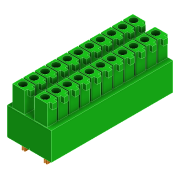
# Autodesk Inventor part: conectores_macho
Saved by Autodesk Inventor 2022 (Build 260153000, 153)
## iProperties
Created: 2022-11-18
Part Number: conectores_macho
Material: Generic
Document SubType Name: Modeling
Designer: ferna
Density: 1 g/cm^3
Appearance: Default
Author: ferna
Autodesk Inventor part; units mm, degrees
ref_plane "YZ Plane" through (0, 0, 0) normal (1, 0, 0) x (0, 1, 0)
ref_plane "XZ Plane" through (0, 0, 0) normal (0, 1, 0) x (-1, 0, 0)
ref_plane "XY Plane" through (0, 0, 0) normal (0, 0, 1) x (1, 0, 0)
sketch "Sketch1" plane through (0, 0, 0) normal (0, 1, 0) x (-1, 0, 0)
  line L0 (-4.4594, 3.5) -> (0, 3.5)
  line L1 (-4.4594, 2.5) -> (-4.4594, 3.5)
  line L2 (-4.6594, 2.5) -> (-4.4594, 2.5)
  line L3 (-4.6594, 2.8) -> (-4.6594, 2.5)
  line L4 (-6, 3.5) -> (-4.6594, 2.8)
  line L5 (-6, 0) -> (-6, 3.5)
  line L6 (-4.6594, 0.7) -> (-6, 0)
  line L7 (-4.6594, 1) -> (-4.6594, 0.7)
  line L8 (-4.4594, 1) -> (-4.6594, 1)
  line L9 (-4.4594, 0) -> (-4.4594, 1)
  line L10 (0, 0) -> (-4.4594, 0)
  line L11 (0, 3.5) -> (0, 0)
  line L12 (0.25, 0) -> (1.75, 0)
  line L13 (1.75, 3.5) -> (1.75, 0)
  line L14 (1.75, 3.5) -> (0.25, 3.5)
  line L15 (0.25, 0) -> (0.25, 3.5)
  line L16 (-6.25, 43.75) -> (-6.25, -0.25)
  line L17 (-2.2297, 3.75) -> (-6.25, 3.75)
  constraints: 36 end point, 1 perpendicular, 1 point on line
extrude "Extrusion1" add sketch "Sketch1" along normal blind 7.5 contours L0 L11 L10 L9 L8 L7 L6 L5 L4 L3 L2 L1
sketch "Sketch2" plane through (0, 7.5, 0) normal (0, 1, 0) x (1, 0, 0)
  line L0 (0, 0) -> (0, -3.5) projected
  line L1 (0, -1.75) -> (2, -1.75)
  circle A0 centre (2, -1.75) radius 1.3281
  dimension "d2" = 2
  constraints: 2 end point, 1 centre point, 1 coincident, 1 horizontal, 1 midpoint
  measures "d2" distance of L1.start L1.end
extrude "Extrusion2" cut sketch "Sketch2" against normal blind 7.5
sketch "Sketch3" plane through (0, 7.5, 0) normal (0, 1, 0) x (1, 0, 0)
  line L0 (4.6594, -2.5) -> (4.6594, -2.8) projected
  line L1 (4.6594, -2.5) -> (6.5607, -2.5)
  line L2 (6.5607, -2.5) -> (6.5607, -3.7591)
  line L3 (6.5607, -3.7591) -> (4.6594, -3.7591)
  line L4 (4.6594, -3.7591) -> (4.6594, -2.5)
  line L5 (4.6594, -1) -> (4.4594, -1) projected
  line L6 (4.6594, -1) -> (6.277, -1)
  line L7 (6.277, -1) -> (6.277, 0.4256)
  line L8 (6.277, 0.4256) -> (4.6594, 0.4256)
  line L9 (4.6594, 0.4256) -> (4.6594, -1)
  line L10 (5.61, -2.5) -> (6.277, -2.5)
  line L11 (6.277, -2.5) -> (6.277, -1)
  line L12 (6.277, -1) -> (5.61, -1)
  line L13 (5.61, -1) -> (5.61, -2.5)
  point P0 (0, 0)
  constraints: 24 end point, 6 parallel, 3 horizontal, 3 perpendicular, 1 midpoint
extrude "Extrusion3" cut sketch "Sketch3" against normal blind 7.5
sketch "Sketch4" plane through (5.61, 7.5, 2.5) normal (1, 0, 0) x (0, 0, -1)
  line L0 (0, -7.5) -> (0, 0) projected
  line L1 (0, -1.9796) -> (1.6962, -1.9796)
  line L2 (1.6962, -1.9796) -> (1.6962, -7.8428)
  line L3 (1.6962, -7.8428) -> (0, -7.8428)
  line L4 (0, -7.8428) -> (0, -1.9796)
  point P0 (2.5, -7.5)
  constraints: 8 end point, 2 parallel, 1 horizontal, 1 perpendicular, 1 point on line
extrude "Extrusion4" cut sketch "Sketch4" against normal up to surface (1.1506 mm away)
sketch "Sketch5" plane through (0, 0, 0) normal (0, -1, 0) x (1, 0, 0)
  line L0 (6.25, -40.25) -> (6.25, 3.75)
  line L1 (2.2297, -0.25) -> (6.25, -0.25)
  line L2 (-1.75, 0) -> (-1.75, 3.5)
  line L3 (4.4594, 0) -> (0, 0) projected
  line L4 (2.2297, 0) -> (2.2297, -0.25)
  line L5 (6.25, 3.75) -> (-1.75, 3.75)
  line L6 (0, 3.5) -> (4.4594, 3.5) projected
  line L7 (-1.75, 3.75) -> (-1.75, 3.5)
  line L8 (-1.75, 0) -> (-1.75, -0.25)
  line L9 (-1.75, -0.25) -> (2.2297, -0.25)
  dimension "d9" = 0.25
  constraints: 16 end point, 3 perpendicular, 2 point on line, 1 midpoint, 1 parallel, 1 vertical
  measures "d9" distance of L4.start L4.end
extrude "Extrusion5" add sketch "Sketch5" along normal blind 10
sketch "Sketch6" plane through (0, -10, 0) normal (0, -1, 0) x (1, 0, 0)
  line L0 (-1.75, 3.75) -> (-1.75, -0.25) projected
  line L1 (-1.75, -0.25) -> (-1.75, 1.75)
  line L2 (-1.75, 1.75) -> (0.25, 1.75)
  line L3 (0.25, 1.75) -> (4.25, 1.75)
  circle A0 centre (0.25, 1.75) radius 1.35
  line L4 (2.9, 0.4) -> (5.6, 0.4)
  line L5 (5.6, 0.4) -> (5.6, 3.1)
  line L6 (5.6, 3.1) -> (2.9, 3.1)
  line L7 (2.9, 3.1) -> (2.9, 0.4)
  line L8 (2.9, 0.4) -> (5.6, 3.1) construction
  line L9 (5.6, 0.4) -> (2.9, 3.1) construction
  point P0 (0, 0)
  dimension "d12" = 2
  dimension "d13" = 2
  dimension "d14" = 4
  dimension "d15" = 2.7
  dimension "d16" = 2.7
  dimension "d17" = 2.7
  constraints: 18 end point, 3 midpoint, 2 parallel, 2 perpendicular, 1 centre point, 1 coincident, 1 horizontal, 1 point on line
  measures "d12" distance of L0.end L1.end
  measures "d13" distance of L1.end L2.end
  measures "d14" distance of L2.end L3.end
  measures "d15" diameter of A0
  measures "d16" distance of L6.end L5.end
  measures "d17" distance of L5.end L4.end
extrude "Extrusion6" cut sketch "Sketch6" against normal blind 8
sketch "Sketch7" plane through (0, -2, 0) normal (0, -1, 0) x (1, 0, 0)
  line L0 (2.9, 3.1) -> (5.6, 3.1) projected
  line L1 (5.6, 0.4) -> (2.9, 0.4) projected
  line L2 (2.9, 3.1) -> (4.0783, 3.1)
  line L3 (4.0783, 3.1) -> (4.0783, 0.4)
  line L4 (4.0783, 0.4) -> (2.9, 0.4)
  line L5 (2.9, 0.4) -> (2.9, 3.1)
  point P0 (0, 0)
  constraints: 8 end point, 2 parallel, 1 horizontal, 1 perpendicular, 1 point on line
extrude "Extrusion7" add sketch "Sketch7" along normal blind 9 separate body
sketch "Sketch8" plane through (0, -11, 0) normal (0, -1, 0) x (1, 0, 0)
  line L0 (4.0783, 0.4) -> (4.0783, 3.1) projected
  line L1 (5.6, 0.4) -> (2.9, 0.4) projected
  line L2 (4.0783, 3.1) -> (3.6783, 3.1)
  line L3 (3.6783, 3.1) -> (3.6783, 0.4)
  line L4 (3.6783, 0.4) -> (4.0783, 0.4)
  line L5 (4.0783, 0.4) -> (4.0783, 3.1)
  line L6 (2.9, 3.1) -> (5.6, 3.1) projected
  line L7 (2.9, 3.1) -> (3.3, 3.1)
  line L8 (3.3, 3.1) -> (3.3, 0.4)
  line L9 (3.3, 0.4) -> (2.9, 0.4)
  line L10 (2.9, 0.4) -> (2.9, 3.1)
  point P0 (0, 0)
  dimension "d22" = 0.4
  dimension "d23" = 0.4
  constraints: 16 end point, 4 parallel, 2 horizontal, 2 perpendicular, 2 point on line
  measures "d22" distance of L4.end L3.end
  measures "d23" distance of L8.end L9.end
extrude "Extrusion8" add sketch "Sketch8" along normal blind 1 contours L1 L3 L2 L0 | L1 L10 L6 L8 bodies 2
fillet "Fillet1" radius 0.5 1 edges at (-1.75, -10, 1.75)
pattern_linear "Rectangular Pattern1" count 11 spacing 4 along (0, 0, 1) count 2 spacing 8 along (1, 0, 0) bodies 1
pattern_linear "Rectangular Pattern2" count 11 spacing 4 along (0, 0, 1) count 2 spacing 8 along (1, 0, 0) bodies 2
sketch "Sketch9" plane through (6.75, -10, -0.25) normal (0, -1, 0) x (1, 0, 0)
  circle A0 centre (1.5, 2) radius 1.35 projected
sketch "Sketch10" plane through (6.75, -10, -0.25) normal (0, -1, 0) x (1, 0, 0)
  circle A0 centre (1.5, 10) radius 1.35 projected
sketch "Sketch11" plane through (6.75, -10, -0.25) normal (0, -1, 0) x (1, 0, 0)
  circle A0 centre (1.5, 14) radius 1.35 projected
sketch "Sketch12" plane through (6.75, -10, -0.25) normal (0, -1, 0) x (1, 0, 0)
  circle A0 centre (1.5, 6) radius 1.35 projected
body "Solid1"
body "Solid2"
